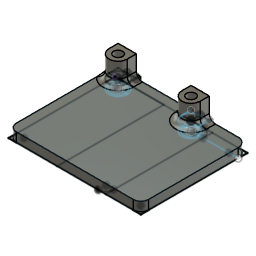
UlTi_PCB_cover (Autodesk Fusion 360 design; units mm, degrees)
Autodesk Fusion 360 part; units mm, degrees
note: some values were not read from the file. Set by a fixed rule: which sketch regions a step uses.
sketch "Sketch1" plane through (0, 0, 0) normal (0, 1, 0) x (1, 0, 0)
  line L0 (0, 0) -> (32, 0)
  line L1 (32, 0) -> (32, -35)
  line L2 (32, -35) -> (0, -35)
  line L3 (0, -35) -> (0, 0)
  line L4 (0, 0) -> (2.5, 0)
  line L5 (0, 0) -> (16, 0)
  line L6 (16, 0) -> (16, -35)
  line L7 (2.5, -3) -> (4, -3)
  circle A0 centre (4, -3) radius 1.5
  line L8 (0, 0) -> (0, -3)
  line L9 (0, 0) -> (2.5, 0)
  arc A1 (2.5, 0) -> (0, -3) centre (3.05, -3) ccw
  circle A2 centre (4, -3) radius 2.4
  line L10 (0, -35) -> (0, -32.5)
  line L11 (0, -35) -> (2.5, -35)
  arc A3 (0, -32.5) -> (2.5, -35) centre (2.5, -32.5) ccw
  arc A4 (29.5, -35) -> (32, -32.5) centre (29.5, -32.5) ccw
  arc A5 (32, -3) -> (29.5, 0) centre (28.95, -3) ccw
  circle A6 centre (28, -3) radius 1.5
  circle A7 centre (28, -3) radius 2.4
  line L12 (28, -3) -> (29.5, -3)
  line L13 (29.5, -3) -> (43.5, -3)
  line L14 (32, 0) -> (43.5, 0)
  line L15 (32, -35) -> (43.5, -35)
  line L16 (43.5, -35) -> (43.5, 0)
  line L17 (43.5, 0) -> (41, 0)
  line L18 (43.5, 0) -> (43.5, -3)
  arc A8 (43.5, -3) -> (41, 0) centre (40.45, -3) ccw
  line L19 (43.5, -35) -> (41, -35)
  line L20 (43.5, -35) -> (43.5, -32.5)
  arc A9 (41, -35) -> (43.5, -32.5) centre (41, -32.5) ccw
  circle A10 centre (4, -3) radius 3
  circle A11 centre (28, -3) radius 3
  dimension "d1" = 32
  dimension "d2" = 35
  dimension "d4" = 2.5
  dimension "d7" = 1.5
  dimension "d8" = 3
  dimension "d9" = 3
  dimension "d10" = 2.5
  dimension "d11" = 4.8
  dimension "d12" = 2.5
  dimension "d13" = 2.5
  dimension "d14" = 14
  dimension "d15" = 11.5
  dimension "d16" = 11.5
  dimension "d17" = 11.5
  dimension "d18" = 2.5
  dimension "d19" = 3
  dimension "d20" = 2.5
  dimension "d21" = 2.5
  dimension "d30" = 0.9
  constraint horizontal L0
  constraint vertical L1
  constraint horizontal L2
  constraint vertical L3
  constraint coincident L0.start L3.end
  constraint perpendicular L3 L4
  constraint midpoint L0 L5.end
  constraint midpoint L2 L6.end
  constraint coincident L7.end A0.centre
  constraint perpendicular L5 L8
  constraint horizontal L9
  constraint tangent L8 A1
  constraint concentric A0 A2
  constraint perpendicular L2 L10
  constraint perpendicular L10 L11
  constraint tangent L10 A3
  constraint symmetric L6 A0 A6
  constraint symmetric L6 L8.end A5.start
  constraint symmetric L6 L4.end A5.end
  constraint symmetric L6 A1 A5
  constraint symmetric L6 A2 A7
  constraint symmetric L6 L10.end A4.end
  constraint symmetric L6 L11.end A4.start
  constraint symmetric L6 A3 A4
  constraint coincident A6.centre A7.centre
  constraint coincident A6 L12.end
  constraint perpendicular L1 L12
  constraint parallel L12 L13
  constraint perpendicular L1 L14
  constraint perpendicular L1 L15
  constraint perpendicular L16 L17
  constraint perpendicular L14 L18
  constraint tangent L16 A8
  constraint perpendicular L16 L19
  constraint perpendicular L19 L20
  constraint tangent L15 A9
  constraint concentric A2 A10
  constraint tangent L0 A10
  constraint concentric A7 A11
  constraint tangent L0 A11
  measures "d1" distance of L0.start L0.end
  measures "d2" distance of L0.start L2.end
  measures "d4" distance of L0.start L4.end
  measures "d7" distance of L7.start L7.end
  measures "d8" diameter of A0
  measures "d9" distance of L0.start L8.end
  measures "d10" distance of L0.start L4.end
  measures "d11" diameter of A2
  measures "d12" distance of L2.end L10.end
  measures "d13" distance of L2.end L11.end
  measures "d14" distance of L12.end L13.end
  measures "d15" distance of A5.start L13.end
  measures "d16" distance of L0.end L14.end
  measures "d17" distance of L1.end L15.end
  measures "d18" distance of L14.end L17.end
  measures "d19" distance of L14.end L13.end
  measures "d20" distance of L15.end L19.end
  measures "d21" distance of L15.end L20.end
  measures "d30" distance of A0 A2
extrude "Extrude4" add sketch "Sketch1" along normal blind 3 contours L0 L2 L3 L5 L6 A1 A3 | L0 L1 L2 L6 A4 L13 A11 | L0 A5 L13 A11 | L0 L1 A5 | L1 L2 A4 | L1 L13 L14 A8 | L1 L13 L15 L16 A9
extrude "Extrude5" add sketch "Sketch1" along normal blind 10 contours A10 | A11 | A2 | A7
sketch "Sketch2" plane through (0, 3, 0) normal (0, 1, 0) x (-1, 0, 0)
  arc A0 (-2.5, 0) -> (0, 3) centre (-3.05, 3) ccw
  line L0 (0, 3) -> (0, 32.5)
  arc A1 (0, 32.5) -> (-2.5, 35) centre (-2.5, 32.5) ccw
  line L1 (-2.5, 35) -> (-41, 35)
  arc A2 (-41, 35) -> (-43.5, 32.5) centre (-41, 32.5) ccw
  line L2 (-43.5, 32.5) -> (-43.5, 3)
  arc A3 (-43.5, 3) -> (-41, 0) centre (-40.45, 3) ccw
  line L3 (-41, 0) -> (-28, 0)
  circle A4 centre (-28, 3) radius 3
  line L4 (-28, 0) -> (-4, 0)
  circle A5 centre (-4, 3) radius 3
  line L5 (-4, 0) -> (-2.5, 0)
  circle A6 centre (-4, 3) radius 3
  line L6 (-4, 3) -> (-1, 3)
  line L7 (-1, 3) -> (-1, 0)
  line L8 (-4, 3) -> (-7, 3)
  line L9 (-7, 3) -> (-7, 0)
  circle A7 centre (-28, 3) radius 3
  line L10 (-28, 3) -> (-25, 3)
  line L11 (-25, 3) -> (-25, 0)
  line L12 (-28, 3) -> (-31, 3)
  line L13 (-31, 3) -> (-31, 0)
  line L14 (-31, 0) -> (-25, 0)
  line L15 (-28, 3) -> (-28, 0)
  line L16 (-4, 3) -> (-4, 0)
  line L17 (-1, 0) -> (-4, 0)
  line L18 (-4, 0) -> (-7, 0)
  dimension "d35" = 6
  dimension "d36" = 3
  constraint concentric A5 A6
  constraint coincident A5.centre A6.centre
  constraint coincident A6 L6.end
  constraint horizontal L6
  constraint perpendicular L6 L7
  constraint coincident A6 L8.end
  constraint perpendicular L7 L8
  constraint coincident L4 L9.end
  constraint tangent A5 L9
  constraint perpendicular L4 L9
  constraint concentric A4 A7
  constraint coincident A4.centre A7.centre
  constraint coincident A7 L10.end
  constraint horizontal L10
  constraint coincident L4 L11.end
  constraint tangent A7 L11
  constraint coincident A7 L12.end
  constraint perpendicular L11 L12
  constraint coincident L3 L13.end
  constraint tangent A7 L13
  constraint coincident L3.end L4.start
  constraint coincident L4.end L5.start
  measures "d35" diameter of A6
  measures "d36" distance of L6.end L7.end
extrude "Extrude6" add sketch "Sketch1" along normal blind 3 contours L0 L3 L4 L5 L8 L9 A1
extrude "Extrude7" add sketch "Sketch2" along normal blind 7 contours A0 A5 L5 A6 L7 L17 | A0 L7 L17 | L4 A5 A6 L9 L18
extrude "Extrude8" add sketch "Sketch2" along normal blind 7 contours A4 L4 A7 L11 L14 | L3 A4 A7 L13 L14
fillet "Fillet2" radius 2 6 edges at (7, 3, 1.5) (4, 3, 6) (1, 3, 1.5) (31, 3, 1.5) (28, 3, 6) (25, 3, 1.5)
